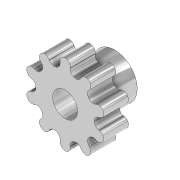
# Autodesk Inventor part: 4th Axis Main Drive Gear
Saved by Autodesk Inventor 2020 (Build 240168000, 168)
## iProperties
Created: 2021-06-28
Part Number: 4th Axis Main Drive Gear
Material: Generic
Document SubType Name: Modeling
Designer: Coy
Density: 1 g/cm^3
Appearance: Chrome - Polished
Author: Coy
Autodesk Inventor part; units mm, degrees
ref_plane "YZ Plane" through (0, 0, 0) normal (1, 0, 0) x (0, 1, 0)
ref_plane "XZ Plane" through (0, 0, 0) normal (0, 1, 0) x (-1, 0, 0)
ref_plane "XY Plane" through (0, 0, 0) normal (0, 0, 1) x (1, 0, 0)
sketch "Sketch4" plane through (0, 0, 0) normal (0, 0, 1) x (1, 0, 0)
  circle A0 centre (0, 0) radius 2.5
  circle A1 centre (0, 0) radius 8.1 construction
  circle A2 centre (0, 0) radius 5.9
  arc A3 (1.0325, 6.8945) -> (-1.044, 6.8927) centre (-0.0059, 7.05) ccw
  arc A4 (-1.7548, 5.633) -> (-1.0289, 6.7927) centre (-2.0671, 6.6355) ccw
  arc A5 (1.0176, 6.7945) -> (1.7454, 5.6359) centre (2.056, 6.6389) ccw
  line L0 (1.0176, 6.7945) -> (1.0325, 6.8945)
  line L1 (-1.0289, 6.7927) -> (-1.044, 6.8927)
  line L2 (0, 0) -> (0, 6.1) construction
  line L3 (-0.0059, 8.1) -> (-0.0059, 9.4985) construction
  arc A6 (-3.2171, 6.1847) -> (-4.8961, 4.9627) centre (-4.1486, 5.7001) ccw
  line L4 (-4.8251, 4.8907) -> (-4.8961, 4.9627)
  arc A7 (-4.7306, 3.5258) -> (-4.8251, 4.8907) centre (-5.5725, 4.1532) ccw
  line L5 (-3.1705, 6.0949) -> (-3.2171, 6.1847)
  arc A8 (-3.1705, 6.0949) -> (-1.9007, 5.5855) centre (-2.239, 6.5795) ccw
  arc A9 (-6.238, 3.1125) -> (-6.878, 1.137) centre (-6.7068, 2.173) ccw
  line L6 (-6.7782, 1.1205) -> (-6.878, 1.137)
  arc A10 (-5.8996, 0.0718) -> (-6.7782, 1.1205) centre (-6.9495, 0.0846) ccw
  line L7 (-6.1475, 3.0674) -> (-6.238, 3.1125)
  arc A11 (-6.1475, 3.0674) -> (-4.8207, 3.4015) centre (-5.6787, 4.0069) ccw
  arc A12 (-6.8761, -1.1485) -> (-6.2328, -3.1229) centre (-6.7031, -2.1842) ccw
  line L8 (-6.1423, -3.0776) -> (-6.2328, -3.1229)
  arc A13 (-4.8151, -3.4096) -> (-6.1423, -3.0776) centre (-5.672, -4.0164) ccw
  line L9 (-6.7763, -1.1319) -> (-6.8761, -1.1485)
  arc A14 (-6.7763, -1.1319) -> (-5.8994, -0.0817) centre (-6.9493, -0.0962) ccw
  arc A15 (-4.8878, -4.9708) -> (-3.2068, -6.19) centre (-4.1391, -5.707) ccw
  line L10 (-3.1603, -6.1002) -> (-3.2068, -6.19)
  arc A16 (-1.8914, -5.5886) -> (-3.1603, -6.1002) centre (-2.228, -6.5832) ccw
  line L11 (-4.8169, -4.8987) -> (-4.8878, -4.9708)
  arc A17 (-4.8169, -4.8987) -> (-4.7247, -3.5337) centre (-5.5656, -4.1625) ccw
  arc A18 (-1.0325, -6.8945) -> (1.044, -6.8927) centre (0.0059, -7.05) ccw
  line L12 (1.0289, -6.7927) -> (1.044, -6.8927)
  arc A19 (1.7548, -5.633) -> (1.0289, -6.7927) centre (2.0671, -6.6355) ccw
  line L13 (-1.0176, -6.7945) -> (-1.0325, -6.8945)
  arc A20 (-1.0176, -6.7945) -> (-1.7454, -5.6359) centre (-2.056, -6.6389) ccw
  arc A21 (3.2171, -6.1847) -> (4.8961, -4.9627) centre (4.1486, -5.7001) ccw
  line L14 (4.8251, -4.8907) -> (4.8961, -4.9627)
  arc A22 (4.7306, -3.5258) -> (4.8251, -4.8907) centre (5.5725, -4.1532) ccw
  line L15 (3.1705, -6.0949) -> (3.2171, -6.1847)
  arc A23 (3.1705, -6.0949) -> (1.9007, -5.5855) centre (2.239, -6.5795) ccw
  arc A24 (6.238, -3.1125) -> (6.878, -1.137) centre (6.7068, -2.173) ccw
  line L16 (6.7782, -1.1205) -> (6.878, -1.137)
  arc A25 (5.8996, -0.0718) -> (6.7782, -1.1205) centre (6.9495, -0.0846) ccw
  line L17 (6.1475, -3.0674) -> (6.238, -3.1125)
  arc A26 (6.1475, -3.0674) -> (4.8207, -3.4015) centre (5.6787, -4.0069) ccw
  arc A27 (6.8761, 1.1485) -> (6.2328, 3.1229) centre (6.7031, 2.1842) ccw
  line L18 (6.1423, 3.0776) -> (6.2328, 3.1229)
  arc A28 (4.8151, 3.4096) -> (6.1423, 3.0776) centre (5.672, 4.0164) ccw
  line L19 (6.7763, 1.1319) -> (6.8761, 1.1485)
  arc A29 (6.7763, 1.1319) -> (5.8994, 0.0817) centre (6.9493, 0.0962) ccw
  arc A30 (4.8878, 4.9708) -> (3.2068, 6.19) centre (4.1391, 5.707) ccw
  line L20 (3.1603, 6.1002) -> (3.2068, 6.19)
  arc A31 (1.8914, 5.5886) -> (3.1603, 6.1002) centre (2.228, 6.5832) ccw
  line L21 (4.8169, 4.8987) -> (4.8878, 4.9708)
  arc A32 (4.8169, 4.8987) -> (4.7247, 3.5337) centre (5.5656, 4.1625) ccw
  point P0 (-4.7658, 6.5496)
  point P1 (-7.7054, 2.4974)
  point P2 (-7.7017, -2.5086)
  point P3 (-4.7563, -6.5565)
  point P4 (0.0059, -8.1)
  point P5 (4.7658, -6.5496)
  point P6 (7.7054, -2.4974)
  point P7 (7.7017, 2.5086)
  point P8 (4.7563, 6.5565)
  point P9 (-4.7306, 3.5258)
  point P10 (-4.8207, 3.4015)
  point P11 (-5.8996, 0.0718)
  point P12 (-5.8994, -0.0817)
  point P13 (-4.8151, -3.4096)
  point P14 (-4.7247, -3.5337)
  point P15 (-1.8914, -5.5886)
  point P16 (-1.7454, -5.6359)
  point P17 (1.7548, -5.633)
  point P18 (1.9007, -5.5855)
  point P19 (4.7306, -3.5258)
  point P20 (4.8207, -3.4015)
  point P21 (5.8996, -0.0718)
  point P22 (5.8994, 0.0817)
  point P23 (4.8151, 3.4096)
  point P24 (4.7247, 3.5337)
  point P25 (1.8914, 5.5886)
  point P26 (-1.9007, 5.5855)
  dimension "d19" = 5
  dimension "d20" = 16.2
  dimension "d21" = 2.2
  dimension "d22" = 2.1
  dimension "d23" = 2.1
  dimension "d24" = 2.1
  dimension "d27" = 360
  constraints: 72 point on circle, 44 end point, 33 centre point, 7 tangent, 2 coincident, 2 line through centre, 2 vertical, 151 other
  measures "d19" diameter of A0
  measures "d20" diameter of A1
  measures "d21" radial gap between concentric circles of A1 A2
  measures "d22" diameter of A3
  measures "d23" diameter of A5
  measures "d24" diameter of A4
extrude "Extrusion4" add sketch "Sketch4" along normal blind 5
sketch "Sketch5" plane through (0, 0, 0) normal (0, 0, -1) x (-1, 0, 0)
  circle A0 centre (0, 0) radius 2.5
  circle A1 centre (0, 0) radius 4.5
  dimension "d31" = 2
  constraints: 2 centre point, 1 coincident
  measures "d31" radial gap between concentric circles of A0 A1
extrude "Extrusion5" add sketch "Sketch5" along normal blind 5
sketch "Sketch6" plane through (0, 0, 0) normal (1, 0, 0) x (0, 1, 0)
  line L0 (4.5, 0) -> (4.5, -5) projected
  line L1 (4.5, -2.5) -> (-4.5, -2.5) construction
  line L2 (-4.5, 0) -> (-4.5, -5) construction
  circle A0 centre (0, -2.5) radius 1
  point P0 (0, 0)
  dimension "d34" = 2
  constraints: 3 midpoint, 2 end point, 1 centre point
  measures "d34" diameter of A0
extrude "Extrusion6" cut sketch "Sketch6" against normal blind 5
equation "\"d23\" = d22"
equation "\"d24\" = d22"
body "Solid2"
